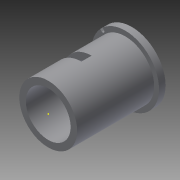
# Autodesk Inventor part: Piston Shaft
Saved by Autodesk Inventor 2015 (Build 190159000, 159)
## iProperties
Created: 2016-02-13
Part Number: Piston Shaft
Material: Generic
Document SubType Name: Modeling
Designer: Owner
Density: 1 g/cm^3
Appearance: Default
Mass: 2.76665 g
Surface Area: 30.1443 cm^2
Volume: 2.76665 cm^3
Author: Owner
Autodesk Inventor part; units mm, degrees
ref_plane "YZ Plane" through (0, 0, 0) normal (1, 0, 0) x (0, 1, 0)
ref_plane "XZ Plane" through (0, 0, 0) normal (0, 1, 0) x (-1, 0, 0)
sketch "Sketch1" plane through (0, 0, 0) normal (0, 0, 1) x (1, 0, 0)
  circle A0 centre (0, 0) radius 10.541
  dimension "d0" = 21.082
  constraints: 1 centre point, 1 coincident
  measures "d0" diameter of A0
extrude "Extrusion1" add sketch "Sketch1" along normal blind 2.032
ref_plane "Work Plane4" through (0, 0, 15.6972) normal (0, 0, -1) x (-1, 0, 0)
sketch "Sketch2" plane through (0, 0, 2.032) normal (0, 0, 1) x (1, 0, 0)
  circle A0 centre (0, 0) radius 9.017
  dimension "d3" = 18.034
  constraints: 1 centre point, 1 coincident
  measures "d3" diameter of A0
extrude "Extrusion2" add sketch "Sketch2" along normal blind 24.003
sketch "Sketch5" plane through (0, 0, 15.6972) normal (0, 0, -1) x (-1, 0, 0)
  line L0 (0, 0) -> (9.017, 0)
  line L1 (9.017, 0) -> (9.017, 9.017)
  line L2 (9.017, 9.017) -> (0, 9.017)
  line L3 (0, 9.017) -> (0, 0)
  dimension "d16" = 9.017
  dimension "d17" = 9.017
  constraints: 8 end point, 2 parallel, 1 horizontal, 1 perpendicular
  measures "d16" distance of L2.end L1.end
  measures "d17" distance of L0.end L1.end
extrude "Extrusion3" cut sketch "Sketch5" along normal blind 3.175
hole "Hole1" at (0, 0, 26.035) direction (0, 0, -1) diameter 13.97 end through all
sketch "Sketch6" plane through (0, 0, 0) normal (0, 0, -1) x (-1, 0, 0)
  line L0 (0, 0) -> (7.629, -6.3585) construction
  line L1 (0, 0) -> (9.9314, 0) construction
  circle A0 centre (7.629, -6.3585) radius 0.508
  line L2 (7.3038, -6.7487) -> (7.7626, -7.1312)
  circle A1 centre (0, 0) radius 10.541 projected
  line L3 (7.9543, -5.9683) -> (8.4131, -6.3507)
  line L4 (0, 0) -> (7.0226, 7.0226)
  line L5 (0, 0) -> (9.9314, 0) construction
  circle A2 centre (7.0226, 7.0226) radius 0.508
  line L6 (6.6671, 7.3855) -> (7.0903, 7.8)
  line L7 (7.378, 6.6597) -> (7.8083, 7.0811)
  line L8 (10.541, 0) -> (10.541, 7.62)
  dimension "d20" = 9.9314
  dimension "d21" = 39.81
  dimension "d22" = 1.016
  dimension "d25" = 9.9314
  dimension "d26" = 45
  dimension "d27" = 1.016
  dimension "d30" = 7.62
  constraints: 18 end point, 9 point on circle, 4 tangent, 3 parallel, 2 centre point, 2 coincident, 2 equal length, 2 horizontal, 1 vertical
  measures "d20" distance of L0.start L0.end
  measures "d21" angle of L0 L1
  measures "d22" diameter of A0
  measures "d25" distance of L0.start L4.end
  measures "d26" angle of L5 L4
  measures "d27" diameter of A2
  measures "d30" distance of L8.start L8.end
extrude "Extrusion5" cut sketch "Sketch6" against normal through all contours A1 L7 A2 L6 | A2
sketch "Sketch7" plane through (0, 0, 26.035) normal (0, 0, 1) x (1, 0, 0)
  point P0 (0, 0)
body "Solid1"
